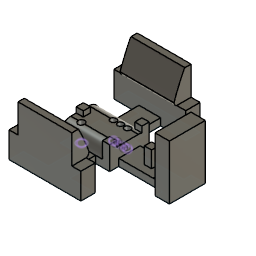
ProgrammingJig (Autodesk Fusion 360 design; units mm, degrees)
part number: 2026-01-31-16-23-09-244
Autodesk Fusion 360 part; units mm, degrees
sketch "Sketch1" plane through (0, 0, 0) normal (0, 0, 1) x (1, 0, 0)
  line L0 (-5.88, -5) -> (-5.88, 0) construction
  line L1 (1.96, -5) -> (1.96, 0) construction
  line L2 (-1.96, -5) -> (-1.96, 0) construction
  line L3 (0, -5) -> (0, 0) construction
  line L4 (-3.92, -5) -> (-3.92, 0) construction
  circle A0 centre (0, 0) radius 0.8125
  circle A1 centre (1.96, 0) radius 0.8625
  circle A2 centre (-1.96, 0) radius 0.8625
  circle A3 centre (-5.88, -5) radius 0.9
  line L5 (17.09, 2.5) -> (21.09, 2.5)
  line L6 (21.09, 2.5) -> (21.09, -7.5)
  line L7 (21.09, -7.5) -> (17.09, -7.5)
  line L8 (17.09, -7.5) -> (17.09, 2.5)
  line L9 (-11.96, 10.1) -> (8.04, 10.1)
  line L10 (8.04, 10.1) -> (8.04, 14.1)
  line L11 (8.04, 14.1) -> (-11.96, 14.1)
  line L12 (-11.96, 14.1) -> (-11.96, 10.1)
  line L13 (-11.96, -15.1) -> (8.04, -15.1)
  line L14 (8.04, -15.1) -> (8.04, -19.1)
  line L15 (8.04, -19.1) -> (-11.96, -19.1)
  line L16 (-11.96, -19.1) -> (-11.96, -15.1)
  line L17 (-8.88, 3) -> (4.96, 3)
  line L18 (4.96, 3) -> (4.96, -8)
  line L19 (4.96, -8) -> (-8.88, -8)
  line L20 (-8.88, -8) -> (-8.88, 3)
  line L21 (-1.96, 3) -> (-1.96, 10.1) construction
  line L22 (4.96, -2.5) -> (17.09, -2.5) construction
  line L23 (-1.96, -15.1) -> (-1.96, -8) construction
  line L24 (4.96, 0.5) -> (17.09, 0.5)
  line L25 (17.09, 0.5) -> (17.09, -5.5)
  line L26 (17.09, -5.5) -> (4.96, -5.5)
  line L27 (4.96, -5.5) -> (4.96, 0.5)
  line L28 (-4.96, 10.1) -> (1.04, 10.1)
  line L29 (1.04, 10.1) -> (1.04, 3)
  line L30 (1.04, 3) -> (-4.96, 3)
  line L31 (-4.96, 3) -> (-4.96, 10.1)
  line L32 (-4.96, -8) -> (1.04, -8)
  line L33 (1.04, -8) -> (1.04, -15.1)
  line L34 (1.04, -15.1) -> (-4.96, -15.1)
  line L35 (-4.96, -15.1) -> (-4.96, -8)
  line L36 (10.0569, -3.4501) -> (12.0569, -3.4501)
  line L37 (12.0569, -3.4501) -> (12.0569, -1.4501)
  line L38 (12.0569, -1.4501) -> (10.0569, -1.4501)
  line L39 (10.0569, -1.4501) -> (10.0569, -3.4501)
  line L40 (4.96, -8) -> (2.96, -8)
  line L41 (2.96, -8) -> (2.96, -6)
  line L42 (2.96, -6) -> (4.96, -6)
  line L43 (4.96, -6) -> (4.96, -8)
  line L44 (4.96, 3) -> (2.96, 3)
  line L45 (2.96, 3) -> (2.96, 1)
  line L46 (2.96, 1) -> (4.96, 1)
  line L47 (4.96, 1) -> (4.96, 3)
  line L48 (-8.88, -3.5) -> (-6.88, -3.5)
  line L49 (-6.88, -3.5) -> (-6.88, -1.5)
  line L50 (-6.88, -1.5) -> (-8.88, -1.5)
  line L51 (-8.88, -1.5) -> (-8.88, -3.5)
  dimension "d3" = 1.96
  dimension "d6" = 1.96
  dimension "d7" = 1.96
  dimension "d8" = 1.96
  dimension "d9" = 1.625
  dimension "d10" = 5
  dimension "d14" = 10.1
  dimension "d15" = 10.1
  dimension "d17" = 3
  dimension "d18" = 3
  dimension "d19" = 3
  dimension "d20" = 3
  dimension "d21" = 4
  dimension "d22" = 4
  dimension "d23" = 4
  dimension "d24" = 3
  dimension "d25" = 3
  dimension "d26" = 3
  dimension "d27" = 3
  dimension "d28" = 20
  dimension "d29" = 10
  dimension "d30" = 20
  dimension "d31" = 6
  dimension "d32" = 6
  dimension "d33" = 6
  dimension "d40" = 2
  dimension "d62" = 1.725
  dimension "d65" = 1.8
  dimension "d66" = 2
  dimension "d67" = 2
  dimension "d68" = 9.05
  constraint coincident L3.end A0.centre
  constraint coincident L1.end A1.centre
  constraint coincident L2.end A2.centre
  constraint equal L0 L4
  constraint equal L2 L4
  constraint equal L2 L3
  constraint equal L1 L3
  constraint coincident L0.start A3.centre
  constraint horizontal L5
  constraint vertical L6
  constraint horizontal L7
  constraint vertical L8
  constraint horizontal L9
  constraint vertical L10
  constraint horizontal L11
  constraint vertical L12
  constraint horizontal L13
  constraint vertical L14
  constraint horizontal L15
  constraint vertical L16
  constraint horizontal L17
  constraint vertical L18
  constraint horizontal L19
  constraint vertical L20
  constraint coincident L17 L21.start
  constraint coincident L9 L21.end
  constraint perpendicular L9 L21
  constraint midpoint L9 L21.end
  constraint midpoint L17 L21.start
  constraint coincident L18 L22.start
  constraint coincident L8 L22.end
  constraint perpendicular L8 L22
  constraint coincident L13 L23.start
  constraint coincident L19 L23.end
  constraint perpendicular L19 L23
  constraint midpoint L19 L23.end
  constraint midpoint L13 L23.start
  constraint midpoint L8 L22.end
  constraint midpoint L18 L22.start
  constraint horizontal L24
  constraint vertical L25
  constraint horizontal L26
  constraint vertical L27
  constraint coincident L8 L25.end
  constraint coincident L18 L24.start
  constraint horizontal L28
  constraint vertical L29
  constraint horizontal L30
  constraint vertical L31
  constraint coincident L17 L29.end
  constraint coincident L9 L28.start
  constraint horizontal L32
  constraint vertical L33
  constraint horizontal L34
  constraint vertical L35
  constraint coincident L13 L33.end
  constraint coincident L19 L32.start
  constraint midpoint L21.end L28
  constraint midpoint L22.end L25
  constraint midpoint L23.end L32
  constraint horizontal L36
  constraint vertical L37
  constraint horizontal L38
  constraint vertical L39
  constraint horizontal L40
  constraint vertical L41
  constraint horizontal L42
  constraint vertical L43
  constraint horizontal L44
  constraint vertical L45
  constraint horizontal L46
  constraint vertical L47
  constraint equal L41 L42
  constraint equal L45 L46
  constraint equal L38 L46
  constraint equal L38 L39
  constraint equal A1 A2
  constraint horizontal L48
  constraint vertical L49
  constraint horizontal L50
  constraint vertical L51
  constraint coincident L20 L48.start
  constraint midpoint L20 L51
  measures "d3" distance of L1 L3
  measures "d6" distance of L2 L3
  measures "d7" distance of L2 L4
  measures "d8" distance of L0 L4
  measures "d9" diameter of A0
  measures "d10" distance of L0.start L0.end
  measures "d14" distance of L3.end L9
  measures "d15" distance of L3.start L13
  measures "d17" distance of L0.end L17
  measures "d18" distance of L0.start L19
  measures "d19" distance of L0.end L20
  measures "d20" distance of L1.end L18
  measures "d21" distance of L9.end L10.end
  measures "d22" distance of L6.end L7.end
  measures "d23" distance of L13.end L14.end
  measures "d24" distance of L4.end L17
  measures "d25" distance of L2.end L17
  measures "d26" distance of L1.end L17
  measures "d27" distance of L3.end L17
  measures "d28" distance of L13.start L13.end
  measures "d29" distance of L5.start L7.end
  measures "d30" distance of L9.start L9.end
  measures "d31" distance of L33 L35
  measures "d32" distance of L24 L26
  measures "d33" distance of L29 L31
  measures "d40" distance of L41.end L42.end
  measures "d62" diameter of A1
  measures "d65" diameter of A3
  measures "d66" distance of L48.start L48.end
  measures "d67" distance of L48.end L49.end
  measures "d68" distance of L8 L10
extrude "Extrude1" add sketch "Sketch1" along normal blind 5 contours L17 L18 L19 L20 L27 L30 L32 L41 L42 L45 L46 L48 L49 L50 | L20 L48 L49 L50 L51 makes body 1
extrude "Extrude2" add sketch "Sketch1" along normal blind 7.2 separate body contours L5 L6 L7 L8 L25 | L9 L10 L11 L12 L28 | L13 L14 L15 L16 L34 makes body 2 at (17.09, -4.1667, 2.4) makes body 3 at (-5.2933, -15.1, 2.4) makes body 4 at (-5.2933, 10.1, 4.8)
extrude "Extrude3" add sketch "Sketch1" along normal blind 2 contours L8 L18 L24 L25 L26 L27 | L9 L17 L28 L29 L30 L31 | L13 L19 L32 L33 L34 L35 bodies 1 2 3 4
extrude "Extrude4" add sketch "Sketch1" along normal blind 6.5 contours L17 L18 L44 L45 L46 L47 | L18 L19 L40 L41 L42 L43 | L20 L48 L49 L50 L51 | L36 L37 L38 L39 bodies 1
sketch "Sketch2" plane through (0, 0, 7.2) normal (0, 0, 1) x (-1, 0, 0)
  line L0 (9.46, -14.1) -> (-5.54, -14.1)
  line L1 (-5.54, -14.1) -> (-5.54, -9.35)
  line L2 (-5.54, -9.35) -> (9.46, -9.35)
  line L3 (9.46, -9.35) -> (9.46, -14.1)
  line L4 (9.46, 19.1) -> (-5.54, 19.1)
  line L5 (-5.54, 19.1) -> (-5.54, 14.35)
  line L6 (-5.54, 14.35) -> (9.46, 14.35)
  line L7 (9.46, 14.35) -> (9.46, 19.1)
  line L8 (11.96, 19.1) -> (-8.04, 19.1)
  line L9 (-8.04, -14.1) -> (11.96, -14.1)
  line L10 (11.96, -10.1) -> (-8.04, -10.1)
  line L11 (-8.04, 15.1) -> (11.96, 15.1)
  dimension "d53" = 15
  dimension "d55" = 15
  dimension "d56" = 0.75
  dimension "d58" = 0.75
  constraint horizontal L0
  constraint vertical L1
  constraint horizontal L2
  constraint vertical L3
  constraint horizontal L4
  constraint vertical L5
  constraint horizontal L6
  constraint vertical L7
  constraint midpoint L4 L8
  constraint midpoint L0 L9
  measures "d53" distance of L1.end L2.end
  measures "d55" distance of L5.end L6.end
  measures "d56" distance of L2 L10
  measures "d58" distance of L6 L11
extrude "Extrude5" add sketch "Sketch2" along normal blind 8 bodies 1
fillet "Fillet1" radius 1 2 edges at (-1.96, -14.35, 7.2) (-1.96, 9.35, 7.2) on bodies 1
fillet "Fillet2" offset 3 second offset 7 tangency weight 0.1 2 edges at (-1.96, 9.35, 15.2) (-1.96, -14.35, 15.2) measured on face at (-4.46, 10.9333, 15.2) measured on face at (-4.46, -15.9333, 15.2) on bodies 1
sketch "Sketch3" plane through (0, 0, 0) normal (0, 0, -1) x (1, 0, 0)
  line L0 (1.04, -3) -> (4.96, -3)
  line L1 (4.96, -3) -> (4.96, -0.5)
  line L2 (4.96, -0.5) -> (17.09, -0.5)
  line L3 (17.09, -0.5) -> (17.09, -2.5)
  line L4 (17.09, -2.5) -> (21.09, -2.5)
  line L5 (21.09, -2.5) -> (21.09, 7.5)
  line L6 (21.09, 7.5) -> (17.09, 7.5)
  line L7 (17.09, 7.5) -> (17.09, 5.5)
  line L8 (17.09, 5.5) -> (4.96, 5.5)
  line L9 (4.96, 5.5) -> (4.96, 8)
  line L10 (4.96, 8) -> (1.04, 8)
  line L11 (1.04, 8) -> (1.04, 15.1)
  line L12 (1.04, 15.1) -> (8.04, 15.1)
  line L13 (8.04, 15.1) -> (8.04, 19.1)
  line L14 (8.04, 19.1) -> (-11.96, 19.1)
  line L15 (-11.96, 19.1) -> (-11.96, 15.1)
  line L16 (-11.96, 15.1) -> (-4.96, 15.1)
  line L17 (-4.96, 15.1) -> (-4.96, 8)
  line L18 (-4.96, 8) -> (-8.88, 8)
  line L19 (-8.88, 8) -> (-8.88, -3)
  line L20 (-8.88, -3) -> (-4.96, -3)
  line L21 (-4.96, -3) -> (-4.96, -10.1)
  line L22 (-4.96, -10.1) -> (-11.96, -10.1)
  line L23 (-11.96, -10.1) -> (-11.96, -14.1)
  line L24 (-11.96, -14.1) -> (8.04, -14.1)
  line L25 (8.04, -14.1) -> (8.04, -10.1)
  line L26 (8.04, -10.1) -> (1.04, -10.1)
  line L27 (1.04, -10.1) -> (1.04, -3)
  circle A0 centre (-5.88, 5) radius 1.25
  circle A1 centre (0, 0) radius 1.25
  circle A2 centre (0, 0) radius 0.8125
  circle A3 centre (1.96, 0) radius 0.8625
  circle A4 centre (-5.88, 5) radius 0.9
  circle A5 centre (-1.96, 0) radius 0.8625
  dimension "d59" = 2.5
  constraint equal A0 A1
  measures "d59" diameter of A0
extrude "Extrude6" cut sketch "Sketch3" against normal blind 1 contours A0 | A1 A3 | A1 A3 A5 | A1 A5 | A2 | A4 picked at (1.1975, -0.0626) picked at (-1.1975, 0) bodies 1
sketch "Sketch4" plane through (0, 0, 0) normal (0, 0, -1) x (1, 0, 0)
  line L0 (1.04, -3) -> (4.96, -3)
  line L1 (4.96, -3) -> (4.96, -0.5)
  line L2 (4.96, -0.5) -> (17.09, -0.5)
  line L3 (17.09, -0.5) -> (17.09, -2.5)
  line L4 (17.09, -2.5) -> (21.09, -2.5)
  line L5 (21.09, -2.5) -> (21.09, 7.5)
  line L6 (21.09, 7.5) -> (17.09, 7.5)
  line L7 (17.09, 7.5) -> (17.09, 5.5)
  line L8 (17.09, 5.5) -> (4.96, 5.5)
  line L9 (4.96, 5.5) -> (4.96, 8)
  line L10 (4.96, 8) -> (1.04, 8)
  line L11 (1.04, 8) -> (1.04, 15.1)
  line L12 (1.04, 15.1) -> (8.04, 15.1)
  line L13 (8.04, 15.1) -> (8.04, 19.1)
  line L14 (8.04, 19.1) -> (-11.96, 19.1)
  line L15 (-11.96, 19.1) -> (-11.96, 15.1)
  line L16 (-11.96, 15.1) -> (-4.96, 15.1)
  line L17 (-4.96, 15.1) -> (-4.96, 8)
  line L18 (-4.96, 8) -> (-8.88, 8)
  line L19 (-8.88, 8) -> (-8.88, -3)
  line L20 (-8.88, -3) -> (-4.96, -3)
  line L21 (-4.96, -3) -> (-4.96, -10.1)
  line L22 (-4.96, -10.1) -> (-11.96, -10.1)
  line L23 (-11.96, -10.1) -> (-11.96, -14.1)
  line L24 (-11.96, -14.1) -> (8.04, -14.1)
  line L25 (8.04, -14.1) -> (8.04, -10.1)
  line L26 (8.04, -10.1) -> (1.04, -10.1)
  line L27 (1.04, -10.1) -> (1.04, -3)
  circle A0 centre (-5.88, 5) radius 1.25
  arc A1 (-1.1888, -0.3863) -> (1.1888, -0.3863) centre (0, 0) ccw
  arc A2 (-1.1888, 0.3863) -> (-1.1888, -0.3863) centre (-1.96, 0) ccw
  arc A3 (1.1888, 0.3863) -> (-1.1888, 0.3863) centre (0, 0) ccw
  arc A4 (1.1888, -0.3863) -> (1.1888, 0.3863) centre (1.96, 0) ccw
fillet "Fillet3" radius 2.5 1 edges at (17.09, -2.5, 2) on bodies 1
extrude "Extrude7" add 1 faces at (18.4233, -4.1667, 7.2) along direction (0, 0, 1) blind 8 on bodies 1 bodies 1
fillet "Fillet4" radius 3 2 edges at (-2.96, -8, 5) (-2.96, 3, 5) on bodies 1
equation "d6 = d3"
equation "d7 = d6"
equation "d8 = d7"
equation "d15 = d14"
equation "d17 = d19"
equation "d18 = d19"
equation "d20 = d19"
equation "d22 = d21"
equation "d23 = d22"
equation "d24 = d17"
equation "d25 = d24"
equation "d26 = d25"
equation "d27 = d19"
equation "d32 = d31"
equation "d33 = d31"
equation "d58 = d56"
equation "d66 = d40"
equation "d67 = d40"
